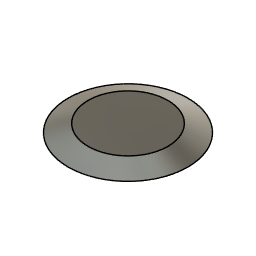
Switch_Floor (Autodesk Fusion 360 design; units mm, degrees)
Autodesk Fusion 360 part; units mm, degrees
sketch "スケッチ3" plane through (0, 0, 0) normal (0, 0, 1) x (1, 0, 0)
  circle A0 centre (0, 0) radius 750
  dimension "d8" = 1500
  constraint coincident A0.centre origin
  measures "d8" diameter of A0
ref_plane "作業平面1" through (0, 0, 100) normal (0, 0, 1) x (1, 0, 0)
sketch "スケッチ6" plane through (0, 0, 100) normal (0, 0, 1) x (1, 0, 0)
  circle A0 centre (0, 0) radius 500
  dimension "d11" = 1000
  constraint coincident A0.centre origin
  measures "d11" diameter of A0
loft "ロフト1" add profiles "スケッチ3", "スケッチ6" section 1 section 2 makes body 1
extrude "押し出し2" cut sketch "スケッチ6" against normal blind 100 bodies 1
extrude "押し出し3" add sketch "スケッチ6" against normal blind 100 separate body makes body 2
named bodies: "ButtonFrame", "Button"
